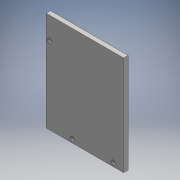
# Autodesk Inventor part: Arduino_Screw_Hole_Base
Saved by Autodesk Inventor 2016 (Build 200138000, 138)
## iProperties
Created: 2018-09-16
Part Number: Arduino_Screw_Hole_Base
Material: Generic
Document SubType Name: Modeling
Designer: Kyle
Density: 1 g/cm^3
Appearance: Default
Author: Kyle
Autodesk Inventor part; units mm, degrees
ref_plane "YZ Plane" through (0, 0, 0) normal (1, 0, 0) x (0, 1, 0)
ref_plane "XZ Plane" through (0, 0, 0) normal (0, 1, 0) x (-1, 0, 0)
ref_plane "XY Plane" through (0, 0, 0) normal (0, 0, 1) x (1, 0, 0)
sketch "Sketch1" plane through (0, 0, 0) normal (0, 1, 0) x (-1, 0, 0)
  line L0 (-26.5, 34) -> (26.5, 34)
  line L1 (26.5, 34) -> (26.5, -34)
  line L2 (26.5, -34) -> (-26.5, -34)
  line L3 (-26.5, -34) -> (-26.5, 34)
  line L4 (-26.5, 34) -> (26.5, -34) construction
  line L5 (26.5, 34) -> (-26.5, -34) construction
  line L6 (26.5, 34) -> (26.5, 19)
  line L7 (-26.5, -34) -> (-19.5, -34)
  line L8 (-26.5, -34) -> (8.5, -34)
  circle A0 centre (8.5, -31.5) radius 1.5
  circle A1 centre (-19.5, -31.5) radius 1.5
  line L9 (-19.5, -33) -> (-19.5, -34)
  line L10 (8.5, -33) -> (8.5, -34)
  circle A2 centre (-19.5, -31.5) radius 1.5
  circle A3 centre (24, 19) radius 1.5
  line L11 (25.5, 19) -> (26.5, 19)
  line L12 (26.5, 19) -> (25.5, 19)
  point P0 (0, 0)
  dimension "d6" = 3
  dimension "d7" = 3
  dimension "d9" = 3
  dimension "d0" = 53
  dimension "d1" = 68
  dimension "d2" = 15
  dimension "d3" = 7
  dimension "d4" = 35
  dimension "d12" = 1
  dimension "d13" = 1
  constraints: 26 end point, 3 equal length, 3 point on line, 2 midpoint, 2 perpendicular, 2 vertical alignment, 1 centre point, 1 coincident, 1 horizontal, 1 horizontal alignment, 1 vertical, 7 other
  measures "d0" distance of L1.end L2.end
  measures "d1" distance of L0.end L1.end
  measures "d2" distance of L0.end L6.end
  measures "d3" distance of L2.end L7.end
  measures "d4" distance of L2.end L8.end
  measures "d12" distance of L10.start L8.end
  measures "d13" distance of L11.start L6.end
sketch "Sketch2" plane through (0, 0, 0) normal (0, 1, 0) x (-1, 0, 0)
  line L0 (0, 0) -> (0, 34)
  line L1 (0, 34) -> (0, 21.5)
  line L2 (0, 21.5) -> (26.5, 21.5)
  line L3 (26.5, 21.5) -> (26.5, -34)
  line L4 (26.5, -34) -> (-22, -34)
  line L5 (-22, -34) -> (-22, 21.5)
  line L6 (-22, 21.5) -> (0, 21.5)
  line L7 (26.5, 21.5) -> (26.5, 16.5)
  line L8 (21.5, 16.5) -> (-22, 16.5)
  line L9 (-22, 16.5) -> (-17, 16.5)
  line L10 (-22, 21.5) -> (-17, 21.5)
  line L11 (-17, 16.5) -> (-17, -29)
  line L12 (-22, -34) -> (-22, -29)
  line L13 (-17, -29) -> (21.5, -29)
  line L14 (26.5, -34) -> (21.5, -34)
  line L15 (21.5, -29) -> (21.5, 16.5)
  circle A0 centre (24, 19) radius 1.5
  line L16 (21.5, -29) -> (8.5, -29)
  line L17 (8.5, -29) -> (8.5, -31.5)
  circle A1 centre (8.5, -31.5) radius 1.5
  circle A2 centre (-19.5, -31.5) radius 1.5
  circle A3 centre (8.5, -31.5) radius 1.5
  line L18 (26.5, 21.5) -> (25.0607, 20.0607)
  line L19 (-17, -29) -> (-18.4393, -30.4393)
  line L20 (-20.5607, -32.5607) -> (-22, -34)
  point P0 (-17, -6.25)
  dimension "d25" = 3
  dimension "d14" = 34
  dimension "d15" = 12.5
  dimension "d16" = 26.5
  dimension "d17" = 55.5
  dimension "d18" = 48.5
  dimension "d19" = 55.5
  dimension "d20" = 5
  dimension "d21" = 48.5
  dimension "d23" = 5
  dimension "d24" = 5
  dimension "d26" = 13
  dimension "d27" = 3
  dimension "d28" = 3
  dimension "d29" = 3
  constraints: 42 end point, 9 point on line, 7 perpendicular, 3 centre point, 2 coincident, 2 horizontal, 2 point on circle, 2 vertical, 1 midpoint, 4 other
  measures "d14" distance of L0.start L0.end
  measures "d15" distance of L0.end L1.end
  measures "d16" distance of L1.end L2.end
  measures "d17" distance of L2.end L3.end
  measures "d18" distance of L3.end L4.end
  measures "d19" distance of L4.end L5.end
  measures "d20" distance of L2.end L7.end
  measures "d21" distance of L7.end L8.end
  measures "d23" distance of L4.end L12.end
  measures "d24" distance of L3.end L14.end
  measures "d26" distance of L13.end L16.end
  measures "d27" diameter of A1
  measures "d28" diameter of A2
  measures "d29" diameter of A3
extrude "Extrusion1" add sketch "Sketch2" along normal blind 4 contours L8 L5 L6 L0 | L0 L2 L3 L4 L20 A2 L19 L13 L15 L8 | L11 L19 A2 L20 L5 L8
extrude "Extrusion2" add sketch "Sketch1" against normal blind 3
body "Solid1"
